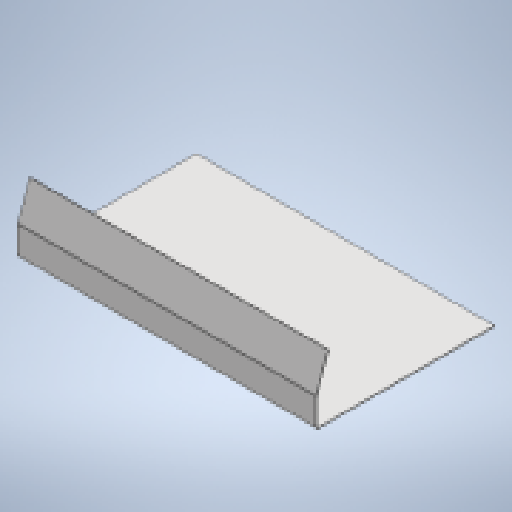
# Autodesk Inventor part: TRM 011 bottom main
Saved by Autodesk Inventor 2025 (Build 290162010, 162A)
## iProperties
Created: 2024-08-07
Part Number: TRM 011 bottom main
Material: AISI 304
Document SubType Name: Sheet Metal
Designer: pokla
Density: 8.02768 g/cm^3
Flat Pattern Width: 65.6279 cm
Flat Pattern Length: 50 cm
Flat Pattern Area: 3281.39 cm^2
Sheet Metal Rule: AISI304 2mm Die16
Sheet Metal Width: 656,279 mm
Sheet Metal Length: 500,000 mm
Sheet Metal Area: 328139,466 mm^2
Appearance: Default
Stock Number: ТРМ 011 дно основное
Author: pokla
Autodesk Inventor part; units mm, degrees
ref_plane "YZ Plane" through (0, 0, 0) normal (1, 0, 0) x (0, 1, 0)
ref_plane "XZ Plane" through (0, 0, 0) normal (0, 1, 0) x (-1, 0, 0)
ref_plane "XY Plane" through (0, 0, 0) normal (0, 0, 1) x (1, 0, 0)
sketch "Sketch1" plane through (0, 0, 0) normal (0, 0, 1) x (1, 0, 0)
  line L0 (-250, -49.2235) -> (250, -49.2235)
  line L1 (250, -49.2235) -> (250, 49.2235)
  line L2 (250, 49.2235) -> (-250, 49.2235)
  line L3 (-250, 49.2235) -> (-250, -49.2235)
  line L4 (-250, -49.2235) -> (250, 49.2235) construction
  line L5 (250, -49.2235) -> (-250, 49.2235) construction
  point P0 (0, 0)
  dimension "d0" = 500
  dimension "d1" = 98.447
  measures "d0" distance of L2.end L1.end
  measures "d1" distance of L1.end L0.end
extrude "Plate1" add sketch "Sketch1" along normal blind 2
sketch "Sketch2" plane through (0, 0, 0) normal (0, 0, -1) x (-1, 0, 0)
  line L0 (-250, 49.2235) -> (250, 49.2235) projected
  line L1 (-250, -49.2235) -> (-250, 49.2235) projected
  line L2 (-230, 29.2235) -> (-30, 29.2235) construction
  line L3 (-30, 29.2235) -> (-30, 9.2235) construction
  line L4 (-30, 9.2235) -> (-230, 9.2235) construction
  line L5 (-230, 9.2235) -> (-230, 29.2235) construction
  point P0 (0, 0)
  dimension "d8" = 200
  dimension "d9" = 20
  dimension "d10" = 20
  dimension "d11" = 20
  constraints: 2 other
  measures "d8" distance of L2.start L2.end
  measures "d9" distance of L2.end L3.end
  measures "d10" distance between parallel lines of L0 L2
  measures "d11" distance between parallel lines of L1 L5
mark "Mark3"
sketch "Sketch3" plane through (250, -47.8093, 1.4142) normal (0, -0.7071068, -0.7071068) x (1, 0, 0)
  line L0 (-500, 0) -> (0, 0)
  line L1 (0, 0) -> (0, 500)
  line L2 (0, 500) -> (-500, 500)
  line L3 (-500, 500) -> (-500, 0)
  constraints: 6 end point, 1 horizontal, 1 perpendicular, 1 vertical
edge flange "Flange1" height 500 angle 45 thickness 2 bend radius 2.75 thickness toward (0, -0.7071068, -0.7071068) relief round relief width 2 relief depth 1 edges at (0, -49.2235, 2) wall of the first edge with corners at (-250, -47.8093, 1.4142) (250, -47.8093, 1.4142) (250, -401.3627, 354.9676) (-250, -401.3627, 354.9676)
bend "Bend1"
corner "Corner1"
sketch "Sketch4" plane through (250, -400.7769, 353.5534) normal (0, -1, 0) x (1, 0, 0)
  line L0 (-500, 0) -> (0, 0)
  line L1 (0, 0) -> (0, 60)
  line L2 (0, 60) -> (-500, 60)
  line L3 (-500, 60) -> (-500, 0)
  constraints: 6 end point, 1 horizontal, 1 perpendicular, 1 vertical
edge flange "Flange2" height 60 angle 45 thickness 2 bend radius 2.75 thickness toward (0, -1, 0) relief round relief width 2 relief depth 1 edges at (0, -401.3627, 354.9676) wall of the first edge with corners at (-250, -400.7769, 353.5534) (250, -400.7769, 353.5534) (250, -400.7769, 413.5534) (-250, -400.7769, 413.5534)
bend "Bend2"
corner "Corner2"
equation "\"d2\" = Thickness"
equation "\"d12\" = BendReliefWidth"
equation "\"d13\" = BendReliefDepth"
equation "\"d14\" = MinimumRemnant"
equation "\"d15\" = TransitionRadius"
equation "\"d18\" = BendRadius"
equation "\"d19\" = CornerReliefSize"
equation "\"d20\" = GapSize"
equation "\"d21\" = JacobiRadiusSize"
equation "\"d22\" = BendReliefWidth"
equation "\"d23\" = BendReliefDepth"
equation "\"d24\" = MinimumRemnant"
equation "\"d25\" = TransitionRadius"
equation "\"d28\" = BendRadius"
equation "\"d29\" = CornerReliefSize"
equation "\"d30\" = GapSize"
equation "\"d31\" = JacobiRadiusSize"
equation "\"BendReliefWidth\" = Thickness"
equation "\"BendReliefDepth\" = 0.5 * Thickness"
equation "\"CornerReliefSize\" = 4 * Thickness"
equation "\"MinimumRemnant\" = 2 * Thickness"
equation "\"TransitionRadius\" = BendRadius"
equation "\"JacobiRadiusSize\" = BendRadius"
equation "\"GapSize\" = Thickness"
equation "\"Thickness\" = 2"
equation "\"BendRadius\" = 2.75"
body "Solid1"
